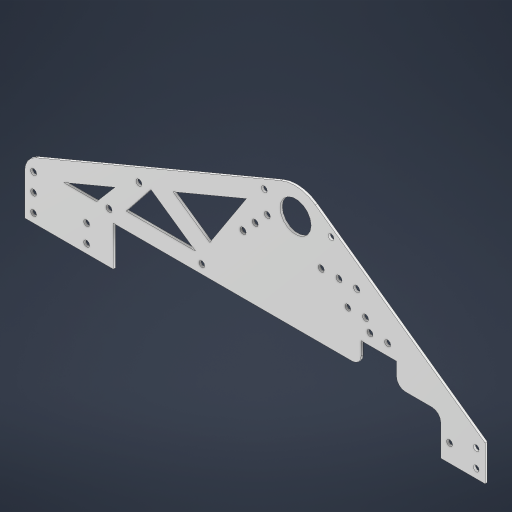
# Autodesk Inventor part: plate_right
Saved by Autodesk Inventor 2024 (Build 280153000, 153)
## iProperties
Created: 2023-11-09
Part Number: plate_right
Material: Acetal Resin, White
Document SubType Name: Modeling
Designer: avere
Density: 1.425 g/cm^3
Appearance: Smooth - White
Author: avere
Autodesk Inventor part; units mm, degrees
ref_plane "YZ Plane" through (0, 0, 0) normal (1, 0, 0) x (0, 1, 0)
ref_plane "XZ Plane" through (0, 0, 0) normal (0, 1, 0) x (-1, 0, 0)
ref_plane "XY Plane" through (0, 0, 0) normal (0, 0, 1) x (1, 0, 0)
sketch "Sketch1" plane through (0, 0, 0) normal (0, 0, 1) x (1, 0, 0)
  circle A0 centre (0, 0) radius 2.0955
  circle A1 centre (0, 12.7) radius 2.0955
  line L0 (-6.35, -6.35) -> (-6.35, 23.3043)
  line L1 (177.4388, 108.8227) -> (1.4386, 35.0162)
  line L2 (323.85, -6.35) -> (323.85, 19.05)
  line L3 (323.85, -6.35) -> (292.1, -6.35)
  line L4 (292.1, -6.35) -> (292.1, 15.875)
  line L5 (57.15, -6.35) -> (57.15, 9.525)
  line L6 (-6.35, -6.35) -> (57.15, -6.35)
  line L7 (292.1, -6.35) -> (323.85, -6.35)
  arc A2 (292.1, 15.875) -> (285.75, 22.225) centre (285.75, 15.875) ccw
  circle A3 centre (317.5, 0) radius 2.0955
  circle A4 centre (317.5, 12.7) radius 2.0955
  line L8 (57.15, 22.225) -> (184.15, 22.225)
  circle A5 centre (0, 25.4) radius 2.1844
  arc A6 (1.4386, 35.0162) -> (-6.35, 23.3043) centre (6.35, 23.3043) ccw
  circle A7 centre (298.45, 6.35) radius 2.0955
  arc A8 (202.0251, 106.0678) -> (177.4388, 108.8227) centre (187.2616, 85.399) ccw
  circle A9 centre (187.9687, 91.7095) radius 11.1125
  line L9 (57.15, -6.35) -> (57.15, 22.225)
  line L10 (260.35, 28.575) -> (260.35, 38.1)
  line L11 (260.35, 38.1) -> (234.95, 38.1)
  line L12 (234.95, 38.1) -> (234.95, 28.575)
  line L13 (184.15, 22.225) -> (228.6, 22.225)
  line L14 (266.7, 22.225) -> (285.75, 22.225)
  arc A10 (228.6, 22.225) -> (234.95, 28.575) centre (228.6, 28.575) ccw
  arc A11 (260.35, 28.575) -> (266.7, 22.225) centre (266.7, 28.575) ccw
  line L15 (45.2425, 29.699) -> (58.3779, 45.1224)
  line L16 (66.4245, 34.39) -> (84.1386, 56.6755)
  line L17 (84.1386, 56.6755) -> (116.0822, 34.39)
  line L18 (100.0585, 63.168) -> (126.3723, 44.8101)
  line L19 (116.0822, 34.39) -> (66.4245, 34.39)
  line L20 (45.2425, 29.699) -> (21.5989, 29.699)
  line L21 (21.5989, 29.699) -> (58.3779, 45.1224)
  line L22 (100.0585, 63.168) -> (152.6862, 85.2376)
  line L23 (126.3723, 44.8101) -> (152.6862, 85.2376)
  circle A12 centre (150.2443, 64.09) radius 2.2479
  circle A13 centre (158.9677, 73.32) radius 2.1844
  circle A14 centre (167.6911, 82.55) radius 2.1844
  circle A15 centre (225.425, 53.975) radius 2.0955
  circle A16 centre (238.125, 53.975) radius 2.1844
  line L24 (323.85, 19.05) -> (292.0829, 41.7408)
  line L25 (323.85, 19.05) -> (202.0251, 106.0678)
  circle A17 centre (241.3, 46.0375) radius 2.1844
  circle A18 centre (254, 46.0375) radius 2.1844
  circle A19 centre (206.375, 68.6706) radius 2.1844
  circle A20 centre (219.075, 68.6706) radius 2.1844
  circle A21 centre (231.775, 68.6706) radius 2.2479
  circle A22 centre (213.3687, 91.7095) radius 2.0955
  circle A23 centre (75.5451, 56.6755) radius 2.1844
  circle A24 centre (54.1023, 29.699) radius 2.1844
  circle A25 centre (38.1, 0) radius 2.0955
  circle A26 centre (38.1, 12.7) radius 2.0955
  circle A27 centre (120.65, 28.575) radius 2.0955
  line L26 (120.65, 28.575) -> (171.1717, 106.1946)
  circle A28 centre (165.5067, 97.4911) radius 2.0955
  point P0 (-6.35, 31.75)
  point P1 (292.1, 22.225)
  point P2 (146.05, 22.225)
  point P3 (82.55, 22.225)
  point P4 (260.35, 22.225)
  point P5 (57.15, 9.525)
  dimension "d8" = 4.191
  dimension "d9" = 4.191
  dimension "d10" = 330.2
  dimension "d11" = 38.1
  dimension "d14" = 31.75
  dimension "d15" = 28.575
  dimension "d16" = 6.35
  dimension "d18" = 4.191
  dimension "d19" = 4.191
  dimension "d22" = 63.5
  dimension "d27" = 4.3688
  dimension "d28" = 12.7
  dimension "d29" = 4.191
  dimension "d30" = 25.4
  dimension "d32" = 22.225
  dimension "d35" = 28.575
  dimension "d37" = 15.875
  dimension "d38" = 6.35
  dimension "d60" = 4.4958
  dimension "d64" = 4.3688
  dimension "d65" = 4.3688
  dimension "d69" = 4.3688
  dimension "d78" = 4.3688
  dimension "d79" = 4.3688
  dimension "d97" = 4.191
  dimension "d98" = 4.3688
  dimension "d99" = 4.3688
  dimension "d100" = 4.191
  dimension "d101" = 4.191
  dimension "d104" = 4.191
  constraints: 54 end point, 29 centre point, 13 tangent, 10 point on circle, 10 point on line, 7 perpendicular, 4 horizontal, 4 vertical, 2 parallel, 1 coincident, 1 equal radius, 4 other
  measures "d8" diameter of A0
  measures "d9" diameter of A1
  measures "d10" distance of L0.start L2.start
  measures "d11" distance of L0.start point (-6.35, 31.75)
  measures "d14" distance of L2.start L3.end
  measures "d15" distance of L3.end point (292.1, 22.225)
  measures "d16" radius of A2
  measures "d18" diameter of A3
  measures "d19" diameter of A4
  measures "d22" distance of L0.start L5.start
  measures "d27" diameter of A5
  measures "d28" radius of A6
  measures "d29" diameter of A7
  measures "d30" radius of A8
  measures "d32" diameter of A9
  measures "d35" distance of L5.start L9.end
  measures "d37" distance of point (260.35, 22.225) L10.end
  measures "d38" radius of A10
  measures "d60" diameter of A12
  measures "d64" diameter of A13
  measures "d65" diameter of A14
  measures "d69" diameter of A16
  measures "d78" diameter of A17
  measures "d79" diameter of A18
  measures "d97" diameter of A22
  measures "d98" diameter of A23
  measures "d99" diameter of A24
  measures "d100" diameter of A25
  measures "d101" diameter of A26
  measures "d104" diameter of A28
extrude "Extrusion1" add sketch "Sketch1" along normal blind 1.5875
body "Solid1"
